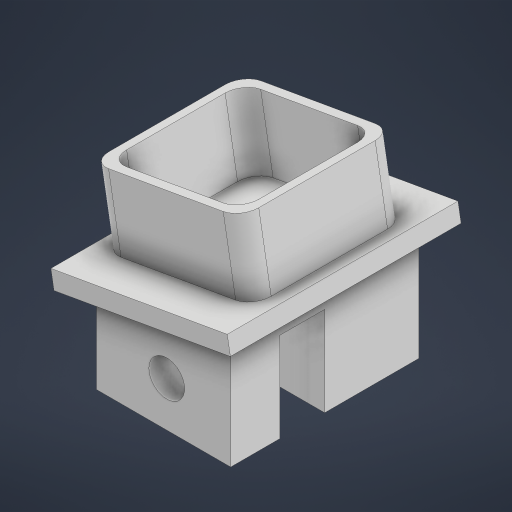
# Autodesk Inventor part: base_75
Saved by Autodesk Inventor 2024 (Build 280153000, 153)
## iProperties
Created: 2023-05-28
Part Number: base_75
Material: Типовые
Document SubType Name: Modeling
Designer: user
Density: 1 g/cm^3
Appearance: По умолчанию
Author: user
Autodesk Inventor part; units mm, degrees
ref_plane "YZ Plane" through (0, 0, 0) normal (1, 0, 0) x (0, 1, 0)
ref_plane "XZ Plane" through (0, 0, 0) normal (0, 1, 0) x (-1, 0, 0)
ref_plane "XY Plane" through (0, 0, 0) normal (0, 0, 1) x (1, 0, 0)
sketch "Эскиз1" plane through (0, 0, 0) normal (0, 0, 1) x (1, 0, 0)
  line L0 (7.5, -5) -> (7.5, 0) projected
  line L1 (5.0577, -5) -> (7.5, -5) projected
  line L2 (5.0577, -5) -> (-4.3392, -5) projected
  line L3 (-6.7815, -5) -> (-4.3392, -5) projected
  line L4 (-6.7815, -5) -> (-6.7815, 0) projected
  line L5 (-6.7815, 0) -> (-4.3392, 0) projected
  line L6 (5.0577, 0) -> (-4.3392, 0) projected
  line L7 (5.0577, 0) -> (7.5, 0) projected
  line L8 (7.5, -10.5) -> (-7.5, -10.5) projected
  line L9 (7.5, 0) -> (-6.7815, 0) projected
  line L10 (7.5, 10.5) -> (7.5, 0) projected
  line L11 (-7.5, 10.5) -> (7.5, 10.5) projected
  line L12 (-7.5, -10.5) -> (-7.5, 10.5) projected
  line L13 (7.5, -10.5) -> (-7.5, -10.5) projected
  line L14 (7.5, -5) -> (7.5, -10.5) projected
  line L15 (7.5, -5) -> (-6.7815, -5) projected
  line L16 (-6.7815, -5) -> (-6.7815, 0) projected
  point P0 (0, 0)
extrude "Выдавливание1" add sketch "Эскиз1" along normal blind 10 contours L14 L8 L12 L11 L10 L7 L6 L5 L4 L3 L2 L1
sketch "Эскиз2" plane through (-7.5, 10.5, 0) normal (0, 1, 0) x (1, 0, 0)
  circle A0 centre (7.8593, -5) radius 2 projected
  point P0 (7.5, 0)
extrude "Выдавливание2" cut sketch "Эскиз2" against normal through all
sketch "Эскиз3" plane through (-7.5, 10.5, 0) normal (0, 1, 0) x (1, 0, 0)
  line L0 (15, -10) -> (0, -10) projected
  line L1 (15, -10) -> (15, -12.6449)
  line L2 (15, -12.6449) -> (0, -10)
  point P0 (7.5, 0)
  dimension "d5" = 10
  constraints: 4 end point, 1 vertical
  measures "d5" angle of L0 L2
extrude "Выдавливание3" add sketch "Эскиз3" against normal up to surface (21 mm away)
sketch "Эскиз4" plane through (7.5, -10.5, 12.6449) normal (-0.1736, 0, 0.9848) x (0.9848, 0, 0.1736)
  line L0 (-15.2314, 0) -> (0, 0) projected
  line L1 (0, 21) -> (0, 0) projected
  line L2 (-15.2314, 21) -> (0, 21) projected
  line L3 (-15.2314, 21) -> (-15.2314, 0) projected
  line L4 (-17.6157, -2.3843) -> (2.3843, -2.3843)
  line L5 (2.3843, -2.3843) -> (2.3843, 23.3843)
  line L6 (2.3843, 23.3843) -> (-17.6157, 23.3843)
  line L7 (-17.6157, 23.3843) -> (-17.6157, -2.3843)
  point P0 (-9.5818, 10.5)
  dimension "d8" = 20
  constraints: 8 end point, 3 other
  measures "d8" distance of L4.start L4.end
extrude "Выдавливание4" add sketch "Эскиз4" along normal blind 2 contours L3 L2 L1 L0 | L7 L6 L5 L4
sketch "Эскиз5" plane through (7.1527, -10.5, 14.6145) normal (-0.1736, 0, 0.9848) x (0.9848, 0, 0.1736)
  line L0 (0.8843, 19) -> (-16.1157, 19)
  line L1 (-16.1157, 19) -> (-16.1157, 2)
  line L2 (-16.1157, 2) -> (0.8843, 2)
  line L3 (0.8843, 2) -> (0.8843, 19)
  line L4 (2.3843, -2.3843) -> (2.3843, 23.3843) projected
  line L5 (-17.6157, -2.3843) -> (2.3843, -2.3843) projected
  line L6 (-0.1157, 18) -> (-15.1157, 18)
  line L7 (-15.1157, 18) -> (-15.1157, 3)
  line L8 (-15.1157, 3) -> (-0.1157, 3)
  line L9 (-0.1157, 3) -> (-0.1157, 18)
  point P0 (-9.5818, 10.5)
  point P1 (0.8843, 10.5)
  point P2 (2.3843, 10.5)
  point P3 (-7.6157, 2)
  point P4 (-7.6157, -2.3843)
  dimension "d11" = 17
  dimension "d12" = 1
  constraints: 16 end point, 4 midpoint, 4 parallel, 3 perpendicular, 1 horizontal, 1 horizontal alignment, 1 vertical alignment, 3 other
  measures "d11" distance of L0.end L1.end
  measures "d12" distance between parallel lines of L3 L9
extrude "Выдавливание5" add sketch "Эскиз5" along normal blind 8
fillet "Сопряжение1" radius 2 8 edges at (7.329, -8.5, 18.7073) (7.329, 8.5, 18.7073) (-9.4128, 8.5, 15.7553) (-9.4128, -8.5, 15.7553) (-8.4279, 7.5, 15.9289) (6.3442, 7.5, 18.5337) (-8.4279, -7.5, 15.9289) (6.3442, -7.5, 18.5337)
equation "\"degg\" = 80deg"
